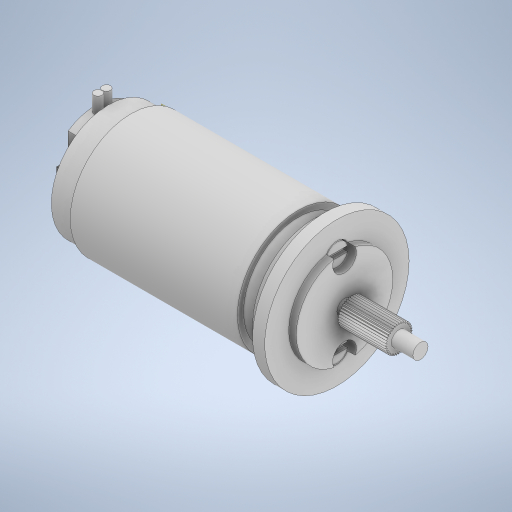
# Autodesk Inventor part: faulhaber_motor
Saved by Autodesk Inventor 2023 (Build 270158000, 158)
## iProperties
Created: 2025-01-11
Part Number: faulhaber_motor
Material: Ogólny
Document SubType Name: Modeling
Designer: kamil
Density: 1 g/cm^3
Appearance: Domyślna
Author: kamil
Autodesk Inventor part; units mm, degrees
ref_plane "YZ Plane" through (0, 0, 0) normal (1, 0, 0) x (0, 1, 0)
ref_plane "XZ Plane" through (0, 0, 0) normal (0, 1, 0) x (-1, 0, 0)
ref_plane "XY Plane" through (0, 0, 0) normal (0, 0, 1) x (1, 0, 0)
sketch "Szkic1" plane through (0, 0, 0) normal (1, 0, 0) x (0, 1, 0)
  circle A0 centre (0, 0) radius 7.5
  dimension "d0" = 15
  constraints: 1 centre point, 1 coincident
  measures "d0" diameter of A0
extrude "Wyciągnięcie proste1" add sketch "Szkic1" along normal blind 3
sketch "Szkic2" plane through (3, 0, 0) normal (1, 0, 0) x (0, 0, -1)
  circle A0 centre (0, 0) radius 8
  dimension "d3" = 16
  constraints: 1 centre point, 1 coincident
  measures "d3" diameter of A0
extrude "Wyciągnięcie proste2" add sketch "Szkic2" along normal blind 22
sketch "Szkic3" plane through (25, 0, 0) normal (1, 0, 0) x (0, 0, -1)
  circle A0 centre (0, 0) radius 7.2
  dimension "d6" = 14.4
  constraints: 1 centre point, 1 coincident
  measures "d6" diameter of A0
extrude "Wyciągnięcie proste3" add sketch "Szkic3" along normal blind 2
sketch "Szkic4" plane through (27, 0, 0) normal (1, 0, 0) x (0, 0, -1)
  circle A0 centre (0, 0) radius 8
  dimension "d9" = 16
  constraints: 1 centre point, 1 coincident
  measures "d9" diameter of A0
extrude "Wyciągnięcie proste4" add sketch "Szkic4" along normal blind 1.5
sketch "Szkic5" plane through (28.5, 0, 0) normal (1, 0, 0) x (0, 0, -1)
  circle A0 centre (0, 0) radius 9.5
  dimension "d12" = 19
  constraints: 1 centre point, 1 coincident
  measures "d12" diameter of A0
extrude "Wyciągnięcie proste5" add sketch "Szkic5" along normal blind 1.6
sketch "Szkic6" plane through (30.1, 0, 0) normal (1, 0, 0) x (0, 0, -1)
  circle A0 centre (0, 0) radius 6.35
  dimension "d15" = 12.7
  constraints: 1 centre point, 1 coincident
  measures "d15" diameter of A0
extrude "Wyciągnięcie proste6" add sketch "Szkic6" along normal blind 1
sketch "Szkic7" plane through (31.1, 0, 0) normal (1, 0, 0) x (0, 0, -1)
  circle A0 centre (0, 0) radius 1
  dimension "d18" = 2
  constraints: 1 centre point, 1 coincident
  measures "d18" diameter of A0
extrude "Wyciągnięcie proste7" add sketch "Szkic7" along normal blind 0.9
sketch "Szkic8" plane through (32, 0, 0) normal (1, 0, 0) x (0, 0, -1)
  circle A0 centre (0, 0) radius 1.8
  dimension "d21" = 3.6
  constraints: 1 centre point, 1 coincident
  measures "d21" diameter of A0
extrude "Wyciągnięcie proste8" add sketch "Szkic8" along normal blind 6.25
sketch "Szkic9" plane through (38.25, 0, 0) normal (1, 0, 0) x (0, 0, -1)
  circle A0 centre (0, 0) radius 1
  dimension "d24" = 2
  constraints: 1 centre point, 1 coincident
  measures "d24" diameter of A0
extrude "Wyciągnięcie proste9" add sketch "Szkic9" along normal blind 2.85
sketch "Szkic10" plane through (0, 0, 0) normal (-1, 0, 0) x (0, 0, 1)
  line L0 (-3.7, 11.8116) -> (3.7, 11.8116)
  line L1 (3.7, 11.8116) -> (3.7, -11.8116)
  line L2 (3.7, -11.8116) -> (-3.7, -11.8116)
  line L3 (-3.7, -11.8116) -> (-3.7, 11.8116)
  line L4 (-3.7, 11.8116) -> (3.7, -11.8116) construction
  line L5 (3.7, 11.8116) -> (-3.7, -11.8116) construction
  circle A0 centre (0, 0) radius 7.5 projected
  circle A1 centre (0, 0) radius 6.7
  point P0 (3.7, 5.5857)
  point P1 (-3.7, 5.5857)
  point P2 (-3.7, -5.5857)
  point P3 (3.7, -5.5857)
  dimension "d27" = 7.4
  dimension "d28" = 0.8
  constraints: 12 end point, 2 midpoint, 2 parallel, 1 centre point, 1 horizontal, 1 perpendicular
  measures "d27" distance of L1.end L2.end
  measures "d28" radial gap between concentric circles of A0 A1
extrude "Wyciągnięcie proste10" add sketch "Szkic10" along normal blind 1.6 contours A1 L1 L3
sketch "Szkic11" plane through (0, 0, 0) normal (-1, 0, 0) x (0, 0, 1)
  line L0 (-3.7, 5.5857) -> (-3.7, -5.5857) projected
  line L1 (3.7, -5.5857) -> (3.7, 5.5857) projected
  line L2 (-2.7, -1.75) -> (-4.7, -1.75)
  line L3 (-4.7, -1.75) -> (-4.7, 1.75)
  line L4 (-4.7, 1.75) -> (-2.7, 1.75)
  line L5 (-2.7, 1.75) -> (-2.7, -1.75)
  line L6 (-2.7, -1.75) -> (-4.7, 1.75) construction
  line L7 (-4.7, -1.75) -> (-2.7, 1.75) construction
  line L8 (2.7, 1.75) -> (4.7, 1.75)
  line L9 (4.7, 1.75) -> (4.7, -1.75)
  line L10 (4.7, -1.75) -> (2.7, -1.75)
  line L11 (2.7, -1.75) -> (2.7, 1.75)
  line L12 (2.7, 1.75) -> (4.7, -1.75) construction
  line L13 (4.7, 1.75) -> (2.7, -1.75) construction
  point P0 (0, 0)
  point P1 (-3.7, 0)
  point P2 (3.7, 0)
  point P3 (3.7, 1.75)
  point P4 (3.7, -1.75)
  point P5 (-3.7, -1.75)
  point P6 (-3.7, 1.75)
  dimension "d31" = 2
  dimension "d32" = 3.5
  dimension "d33" = 2
  dimension "d34" = 3.5
  constraints: 24 end point, 6 midpoint, 4 parallel, 2 horizontal, 2 perpendicular
  measures "d31" distance of L3.end L4.end
  measures "d32" distance of L2.end L3.end
  measures "d33" distance of L9.end L10.end
  measures "d34" distance of L8.end L9.end
extrude "Wyciągnięcie proste11" add sketch "Szkic11" along normal blind 2.1 contours L0 L2 L3 L4 | L1 L8 L9 L10
sketch "Szkic12" plane through (0, 1.75, -3.7) normal (0, 1, 0) x (1, 0, 0)
  line L0 (0, 0) -> (0, -7.4) projected
  line L1 (0, 0) -> (-1.6, 0) projected
  line L2 (-1.6, -7.4) -> (-1.6, 0) projected
  line L3 (0, -7.4) -> (-1.6, -7.4) projected
  circle A0 centre (-0.8, -4.25) radius 0.55
  circle A1 centre (-0.8, -3.15) radius 0.55
  line L4 (-0.8, -3.15) -> (-0.8, -4.25) construction
  line L5 (-1.6, -7.4) -> (0, -7.4) construction
  point P0 (0, -3.7)
  point P1 (-1.6, -3.7)
  point P2 (-0.8, -3.7)
  point P3 (-0.8, -7.4)
  point P4 (-0.8, -3.7)
  dimension "d37" = 1.1
  dimension "d38" = 1.1
  constraints: 3 midpoint, 2 centre point, 2 end point, 2 vertical alignment, 1 equal radius, 1 horizontal alignment, 1 vertical
  measures "d37" diameter of A0
  measures "d38" diameter of A1
extrude "Wyciągnięcie proste12" add sketch "Szkic12" along normal blind 7 contours A0 | A1
sketch "Szkic13" plane through (38.25, 0, 0) normal (1, 0, 0) x (0, 0, -1)
  circle A0 centre (0, 0) radius 1.8 projected
  line L0 (0, 0) -> (0, 1.8)
  line L1 (0, 0) -> (0.3126, 1.7727)
  line L2 (0, 1.8) -> (0.134, 1.5316)
  line L3 (0.134, 1.5316) -> (0.3126, 1.7727)
  dimension "d48" = 10
  dimension "d49" = 0.3
  constraints: 8 end point, 2 point on circle, 1 equal length, 1 vertical
  measures "d48" angle of L0 L1
  measures "d49" distance of L0.end L2.end
extrude "Wyciągnięcie proste13" cut sketch "Szkic13" against normal up to surface (6.25 mm away) contours L3 L2 A0
pattern_circular "Szyk kołowy1" count 36 over 360 about axis through (32, 0, 0) along (1, 0, 0) of "Wyciągnięcie proste13"
sketch "Szkic14" plane through (31.1, 0, 0) normal (1, 0, 0) x (0, 0, -1)
  line L0 (0, -3.9) -> (0, 3.9) construction
  circle A0 centre (0, -5.475) radius 1.575
  circle A1 centre (0, 5.475) radius 1.575
  circle A2 centre (0, 0) radius 6.35 projected
  dimension "d51" = 3.15
  dimension "d52" = 3.15
  dimension "d50" = 7.8
  constraints: 4 vertical alignment, 2 coincident, 2 end point, 1 midpoint, 1 vertical, 4 other
  measures "d50" distance of L0.start L0.end
extrude "Wyciągnięcie proste14" cut sketch "Szkic14" against normal blind 3 contours A0 A2 | A2 A0 | A2 A1 | A1 A2
sketch "Szkic15" plane through (28.1, -5.475, 0) normal (1, 0, 0) x (0, 0, -1)
  circle A0 centre (0, 0) radius 1.575 projected
  circle A1 centre (0, 10.95) radius 1.575 projected
  circle A2 centre (0, 0) radius 1.45
  circle A3 centre (0, 10.95) radius 1.45
  line L0 (1.5, 0.35) -> (-1.5, 0.35)
  line L1 (-1.5, 0.35) -> (-1.5, -0.35)
  line L2 (-1.5, -0.35) -> (1.5, -0.35)
  line L3 (1.5, -0.35) -> (1.5, 0.35)
  circle A4 centre (0, 0) radius 1.575 projected
  line L4 (1.5, 0.35) -> (-1.5, -0.35) construction
  line L5 (-1.5, 0.35) -> (1.5, -0.35) construction
  line L6 (1.5, 11.3) -> (-1.5, 11.3)
  line L7 (-1.5, 11.3) -> (-1.5, 10.6)
  line L8 (-1.5, 10.6) -> (1.5, 10.6)
  line L9 (1.5, 10.6) -> (1.5, 11.3)
  line L10 (1.5, 11.3) -> (-1.5, 10.6) construction
  line L11 (-1.5, 11.3) -> (1.5, 10.6) construction
  point P0 (0, 5.475)
  point P1 (-1.4071, 11.3)
  point P2 (1.4071, 11.3)
  point P3 (1.4071, 10.6)
  point P4 (-1.4071, 10.6)
  point P5 (1.4071, -0.35)
  point P6 (-1.4071, -0.35)
  point P7 (-1.4071, 0.35)
  point P8 (1.4071, 0.35)
  dimension "d55" = 2.9
  dimension "d56" = 2.9
  dimension "d57" = 3
  dimension "d58" = 0.7
  dimension "d59" = 3
  dimension "d60" = 0.7
  constraints: 24 end point, 4 midpoint, 4 parallel, 2 centre point, 2 coincident, 2 horizontal, 2 perpendicular
  measures "d55" diameter of A2
  measures "d56" diameter of A3
  measures "d57" distance of L2.end L1.end
  measures "d58" distance of L1.end L0.end
  measures "d59" distance of L8.end L7.end
  measures "d60" distance of L7.end L6.end
extrude "Wyciągnięcie proste15" add sketch "Szkic15" along normal blind 2 contours L0 A2 | A2 L2 | L6 A3 | A3 L8
extrude "Wyciągnięcie proste16" add sketch "Szkic15" along normal blind 1.5 contours A2 L2 L0 | A3 L8 L6
ref_plane "Płaszczyzna konstrukcyjna1" through (0, -1.75, -9.2) normal (0, 0, -1) x (-1, 0, 0)
sketch "Szkic16" plane through (0, -1.75, -9.2) normal (0, 0, -1) x (-1, 0, 0)
  line L0 (-24.9045, -1.7054) -> (-3.0955, -1.7054) construction
  line L1 (-3.0955, -1.7054) -> (-3.0955, 5.2054) construction
  line L2 (-3.0955, 5.2054) -> (-24.9045, 5.2054) construction
  line L3 (-24.9045, 5.2054) -> (-24.9045, -1.7054) construction
  line L4 (-3, 9.75) -> (-25, 9.75) projected
  line L5 (-21.4558, 2.4542) -> (-22.3793, 2.4542)
  line L6 (-22.3793, 2.4542) -> (-22.3793, 2.0388)
  line L7 (-22.3793, 2.0388) -> (-21.5288, 2.0388)
  line L8 (-21.5288, 2.0388) -> (-21.5288, 1.6199)
  line L9 (-21.5288, 1.6199) -> (-22.3793, 1.6199)
  line L10 (-22.3793, 1.6199) -> (-22.3793, 0.6732)
  line L11 (-22.3793, 0.6732) -> (-22.9284, 0.6732)
  line L12 (-22.9284, 0.6732) -> (-22.9284, 2.8732)
  line L13 (-22.9284, 2.8732) -> (-21.4558, 2.8732)
  line L14 (-21.4558, 2.8732) -> (-21.4558, 2.4542)
  line L15 (-21.4076, 0.6732) -> (-20.6642, 2.8732)
  line L16 (-20.6642, 2.8732) -> (-20.0616, 2.8732)
  line L17 (-20.0616, 2.8732) -> (-19.3182, 0.6732)
  line L18 (-19.3182, 0.6732) -> (-19.8869, 0.6732)
  line L19 (-19.8869, 0.6732) -> (-20.0241, 1.1224)
  line L20 (-20.0241, 1.1224) -> (-20.7159, 1.1224)
  line L21 (-20.7159, 1.1224) -> (-20.8549, 0.6732)
  line L22 (-20.8549, 0.6732) -> (-21.4076, 0.6732)
  line L23 (-20.1454, 1.5218) -> (-20.37, 2.2492)
  line L24 (-20.37, 2.2492) -> (-20.5964, 1.5218)
  line L25 (-20.5964, 1.5218) -> (-20.1454, 1.5218)
  spline S0 degree 2 poles (-18.2092, 0.6268) (-18.6532, 0.6268) (-19.131, 1.0547) (-19.131, 1.4683) knots 0 0 0 1 2 2 2
  line L26 (-19.131, 1.4683) -> (-19.131, 2.8732)
  line L27 (-19.131, 2.8732) -> (-18.5783, 2.8732)
  line L28 (-18.5783, 2.8732) -> (-18.5783, 1.5004)
  spline S1 degree 2 poles (-18.5783, 1.5004) (-18.5783, 1.2704) (-18.4053, 1.0458) (-18.2092, 1.0458) knots 0 0 0 1 2 2 2
  spline S2 degree 2 poles (-18.2092, 1.0458) (-18.0185, 1.0458) (-17.8402, 1.2615) (-17.8402, 1.5004) knots 0 0 0 1 2 2 2
  line L29 (-17.8402, 1.5004) -> (-17.8402, 2.8732)
  line L30 (-17.8402, 2.8732) -> (-17.2875, 2.8732)
  line L31 (-17.2875, 2.8732) -> (-17.2875, 1.4701)
  spline S3 degree 2 poles (-17.2875, 1.4701) (-17.2875, 1.0636) (-17.7528, 0.6268) (-18.2092, 0.6268) knots 0 0 0 1 2 2 2
  line L32 (-15.3959, 0.6732) -> (-16.8632, 0.6732)
  line L33 (-16.8632, 0.6732) -> (-16.8632, 2.8732)
  line L34 (-16.8632, 2.8732) -> (-16.3105, 2.8732)
  line L35 (-16.3105, 2.8732) -> (-16.3105, 1.0921)
  line L36 (-16.3105, 1.0921) -> (-15.3959, 1.0921)
  line L37 (-15.3959, 1.0921) -> (-15.3959, 0.6732)
  line L38 (-13.2762, 0.6732) -> (-13.8288, 0.6732)
  line L39 (-13.8288, 0.6732) -> (-13.8288, 1.6484)
  line L40 (-13.8288, 1.6484) -> (-14.5794, 1.6484)
  line L41 (-14.5794, 1.6484) -> (-14.5794, 0.6732)
  line L42 (-14.5794, 0.6732) -> (-15.1321, 0.6732)
  line L43 (-15.1321, 0.6732) -> (-15.1321, 2.8732)
  line L44 (-15.1321, 2.8732) -> (-14.5794, 2.8732)
  line L45 (-14.5794, 2.8732) -> (-14.5794, 2.0673)
  line L46 (-14.5794, 2.0673) -> (-13.8288, 2.0673)
  line L47 (-13.8288, 2.0673) -> (-13.8288, 2.8732)
  line L48 (-13.8288, 2.8732) -> (-13.2762, 2.8732)
  line L49 (-13.2762, 2.8732) -> (-13.2762, 0.6732)
  line L50 (-13.0569, 0.6732) -> (-12.3135, 2.8732)
  line L51 (-12.3135, 2.8732) -> (-11.7109, 2.8732)
  line L52 (-11.7109, 2.8732) -> (-10.9674, 0.6732)
  line L53 (-10.9674, 0.6732) -> (-11.5361, 0.6732)
  line L54 (-11.5361, 0.6732) -> (-11.6734, 1.1224)
  line L55 (-11.6734, 1.1224) -> (-12.3652, 1.1224)
  line L56 (-12.3652, 1.1224) -> (-12.5042, 0.6732)
  line L57 (-12.5042, 0.6732) -> (-13.0569, 0.6732)
  line L58 (-11.7947, 1.5218) -> (-12.0193, 2.2492)
  line L59 (-12.0193, 2.2492) -> (-12.2457, 1.5218)
  line L60 (-12.2457, 1.5218) -> (-11.7947, 1.5218)
  spline S4 degree 2 poles (-8.9903, 1.3471) (-8.9903, 1.1831) (-9.1151, 0.9353) (-9.2185, 0.8532) knots 0 0 0 1 2 2 2
  spline S5 degree 2 poles (-9.2185, 0.8532) (-9.3433, 0.7552) (-9.6392, 0.6732) (-9.8692, 0.6732) knots 0 0 0 1 2 2 2
  line L61 (-9.8692, 0.6732) -> (-10.7481, 0.6732)
  line L62 (-10.7481, 0.6732) -> (-10.7481, 2.8732)
  line L63 (-10.7481, 2.8732) -> (-9.9726, 2.8732)
  spline S6 degree 2 poles (-9.9726, 2.8732) (-9.7301, 2.8732) (-9.4806, 2.8357) (-9.3718, 2.7769) knots 0 0 0 1 2 2 2
  spline S7 degree 2 poles (-9.3718, 2.7769) (-9.2524, 2.7145) (-9.1365, 2.5006) (-9.1365, 2.3615) knots 0 0 0 1 2 2 2
  spline S8 degree 2 poles (-9.1365, 2.3615) (-9.1365, 2.2011) (-9.2969, 1.9497) (-9.4395, 1.8908) knots 0 0 0 1 2 2 2
  line L64 (-9.4395, 1.8908) -> (-9.4395, 1.8801)
  spline S9 degree 2 poles (-9.4395, 1.8801) (-9.2345, 1.8374) (-8.9903, 1.5717) (-8.9903, 1.3471) knots 0 0 0 1 2 2 2
  spline S10 degree 2 poles (-9.5608, 1.356) (-9.5608, 1.4594) (-9.6428, 1.5753) (-9.7248, 1.6056) knots 0 0 0 1 2 2 2
  spline S11 degree 2 poles (-9.7248, 1.6056) (-9.7747, 1.6252) (-9.9512, 1.6288) (-10.0974, 1.6288) knots 0 0 0 1 2 2 2
  line L65 (-10.0974, 1.6288) -> (-10.199, 1.6288)
  line L66 (-10.199, 1.6288) -> (-10.199, 1.0743)
  line L67 (-10.199, 1.0743) -> (-10.1687, 1.0743)
  spline S12 degree 2 poles (-10.1687, 1.0743) (-9.9548, 1.0743) (-9.7908, 1.0797) (-9.7052, 1.1171) knots 0 0 0 1 2 2 2
  spline S13 degree 2 poles (-9.7052, 1.1171) (-9.6303, 1.151) (-9.5608, 1.2758) (-9.5608, 1.356) knots 0 0 0 1 2 2 2
  spline S14 degree 2 poles (-9.6981, 2.2528) (-9.6981, 2.3062) (-9.7533, 2.4186) (-9.8104, 2.4435) knots 0 0 0 1 2 2 2
  spline S15 degree 2 poles (-9.8104, 2.4435) (-9.8639, 2.4685) (-10.0136, 2.472) (-10.1616, 2.472) knots 0 0 0 1 2 2 2
  line L68 (-10.1616, 2.472) -> (-10.199, 2.472)
  line L69 (-10.199, 2.472) -> (-10.199, 2.0049)
  line L70 (-10.199, 2.0049) -> (-10.1295, 2.0049)
  spline S16 degree 2 poles (-10.1295, 2.0049) (-9.9887, 2.0049) (-9.8746, 2.0103) (-9.8139, 2.0388) knots 0 0 0 1 2 2 2
  spline S17 degree 2 poles (-9.8139, 2.0388) (-9.748, 2.0709) (-9.6981, 2.1797) (-9.6981, 2.2528) knots 0 0 0 1 2 2 2
  line L71 (-8.6729, 0.6732) -> (-8.6729, 2.8732)
  line L72 (-8.6729, 2.8732) -> (-7.1861, 2.8732)
  line L73 (-7.1861, 2.8732) -> (-7.1861, 2.4542)
  line L74 (-7.1861, 2.4542) -> (-8.1238, 2.4542)
  line L75 (-8.1238, 2.4542) -> (-8.1238, 2.0673)
  line L76 (-8.1238, 2.0673) -> (-7.2592, 2.0673)
  line L77 (-7.2592, 2.0673) -> (-7.2592, 1.6484)
  line L78 (-7.2592, 1.6484) -> (-8.1238, 1.6484)
  line L79 (-8.1238, 1.6484) -> (-8.1238, 1.0921)
  line L80 (-8.1238, 1.0921) -> (-7.1861, 1.0921)
  line L81 (-7.1861, 1.0921) -> (-7.1861, 0.6732)
  line L82 (-7.1861, 0.6732) -> (-8.6729, 0.6732)
  line L83 (-4.7793, 0.6732) -> (-5.4514, 0.6732)
  line L84 (-5.4514, 0.6732) -> (-6.0629, 1.4808)
  line L85 (-6.0629, 1.4808) -> (-6.2626, 1.4808)
  line L86 (-6.2626, 1.4808) -> (-6.2626, 0.6732)
  line L87 (-6.2626, 0.6732) -> (-6.8117, 0.6732)
  line L88 (-6.8117, 0.6732) -> (-6.8117, 2.8732)
  line L89 (-6.8117, 2.8732) -> (-5.9274, 2.8732)
  spline S18 degree 2 poles (-5.9274, 2.8732) (-5.7438, 2.8732) (-5.4728, 2.8268) (-5.3569, 2.7555) knots 0 0 0 1 2 2 2
  spline S19 degree 2 poles (-5.3569, 2.7555) (-5.2392, 2.6806) (-5.1002, 2.4471) (-5.1002, 2.2688) knots 0 0 0 1 2 2 2
  spline S20 degree 2 poles (-5.1002, 2.2688) (-5.1002, 2.0174) (-5.3284, 1.7019) (-5.5191, 1.6092) knots 0 0 0 1 2 2 2
  line L90 (-5.5191, 1.6092) -> (-4.7793, 0.6732)
  spline S21 degree 2 poles (-5.6671, 2.1993) (-5.6671, 2.2831) (-5.7313, 2.4025) (-5.8044, 2.4346) knots 0 0 0 1 2 2 2
  spline S22 degree 2 poles (-5.8044, 2.4346) (-5.8561, 2.456) (-5.9827, 2.4685) (-6.0771, 2.4685) knots 0 0 0 1 2 2 2
  line L91 (-6.0771, 2.4685) -> (-6.2626, 2.4685)
  line L92 (-6.2626, 2.4685) -> (-6.2626, 1.8766)
  line L93 (-6.2626, 1.8766) -> (-6.1039, 1.8766)
  spline S23 degree 2 poles (-6.1039, 1.8766) (-5.9898, 1.8766) (-5.8276, 1.9051) (-5.7723, 1.9497) knots 0 0 0 1 2 2 2
  spline S24 degree 2 poles (-5.7723, 1.9497) (-5.7188, 1.9925) (-5.6671, 2.1066) (-5.6671, 2.1993) knots 0 0 0 1 2 2 2
  point P0 (0, 1.75)
  point P1 (-24.9045, 1.75)
  point P2 (-14, 9.75)
  point P3 (-14, 5.2054)
  constraints: 3 midpoint, 1 horizontal alignment, 1 vertical alignment, 2 other
extrude "Wyciągnięcie proste17" cut sketch "Szkic16" against normal blind 1.5
